Autodesk Inventor part; units mm, degrees
(part 2 of 2)
sketch "Sketch10" plane through (0, 0, 10) normal (0, 0, 1) x (1, 0, 0)
  arc A0 (18.6863, 97.4304) -> (17.9083, 97.5423) centre (18.2533, 97.1804) ccw projected
  line L0 (18.6863, 97.4304) -> (19.3213, 96.3305) projected
  arc A1 (19.3213, 96.3305) -> (21.9194, 97.8305) centre (20.6203, 97.0805) ccw projected
  line L1 (21.9194, 97.8305) -> (20.5344, 100.2294) projected
  line L2 (17.725, 88.9676) -> (14.955, 88.9676) projected
  arc A2 (14.955, 89.9676) -> (14.955, 88.9676) centre (14.955, 89.4676) ccw projected
  line L3 (14.955, 89.9676) -> (16.225, 89.9676) projected
  arc A3 (16.225, 89.9676) -> (17.6107, 92.0419) centre (16.225, 91.4676) ccw projected
  line L4 (19.6683, 99.7294) -> (21.0533, 97.3305) projected
  arc A4 (20.1873, 96.8305) -> (21.0533, 97.3305) centre (20.6203, 97.0805) ccw projected
  line L5 (20.1873, 96.8305) -> (19.5523, 97.9304) projected
  arc A5 (19.5523, 97.9304) -> (17.063, 98.0932) centre (18.2533, 97.1804) ccw projected
  arc A6 (11.8587, 96.3305) -> (12.1508, 95.6008) centre (12.2917, 96.0805) ccw projected
  line L6 (11.8587, 96.3305) -> (12.4937, 97.4304) projected
  arc A7 (12.4937, 97.4304) -> (9.8956, 98.9304) centre (11.1947, 98.1804) ccw projected
  line L7 (9.8956, 98.9304) -> (8.5106, 96.5315) projected
  arc A8 (16.225, 90.9676) -> (16.7109, 91.5854) centre (16.225, 91.4676) ccw projected
  line L8 (16.225, 90.9676) -> (14.955, 90.9676) projected
  arc A9 (14.955, 90.9676) -> (14.955, 87.9676) centre (14.955, 89.4676) ccw projected
  line L9 (14.955, 87.9676) -> (17.725, 87.9676) projected
  line L10 (9.3767, 96.0315) -> (10.7617, 98.4304) projected
  arc A10 (11.6277, 97.9304) -> (10.7617, 98.4304) centre (11.1947, 98.1804) ccw projected
  line L11 (11.6277, 97.9304) -> (10.9927, 96.8305) projected
  arc A11 (10.9927, 96.8305) -> (12.0963, 94.5933) centre (12.2917, 96.0805) ccw projected
  arc A12 (37.3863, 97.4304) -> (36.6083, 97.5423) centre (36.9533, 97.1804) ccw projected
  line L12 (37.3863, 97.4304) -> (38.0213, 96.3305) projected
  arc A13 (38.0213, 96.3305) -> (40.6194, 97.8305) centre (39.3203, 97.0805) ccw projected
  line L13 (40.6194, 97.8305) -> (39.2344, 100.2294) projected
  line L14 (36.425, 88.9676) -> (33.655, 88.9676) projected
  arc A14 (33.655, 89.9676) -> (33.655, 88.9676) centre (33.655, 89.4676) ccw projected
  line L15 (33.655, 89.9676) -> (34.925, 89.9676) projected
  arc A15 (34.925, 89.9676) -> (36.3107, 92.0419) centre (34.925, 91.4676) ccw projected
  line L16 (38.3683, 99.7294) -> (39.7533, 97.3305) projected
  arc A16 (38.8873, 96.8305) -> (39.7533, 97.3305) centre (39.3203, 97.0805) ccw projected
  line L17 (38.8873, 96.8305) -> (38.2523, 97.9304) projected
  arc A17 (38.2523, 97.9304) -> (35.763, 98.0932) centre (36.9533, 97.1804) ccw projected
  arc A18 (30.5587, 96.3305) -> (30.8508, 95.6008) centre (30.9917, 96.0805) ccw projected
  line L18 (30.5587, 96.3305) -> (31.1937, 97.4304) projected
  arc A19 (31.1937, 97.4304) -> (28.5956, 98.9304) centre (29.8947, 98.1804) ccw projected
  line L19 (28.5956, 98.9304) -> (27.2106, 96.5315) projected
  arc A20 (34.925, 90.9676) -> (35.4109, 91.5854) centre (34.925, 91.4676) ccw projected
  line L20 (34.925, 90.9676) -> (33.655, 90.9676) projected
  arc A21 (33.655, 90.9676) -> (33.655, 87.9676) centre (33.655, 89.4676) ccw projected
  line L21 (33.655, 87.9676) -> (36.425, 87.9676) projected
  line L22 (28.0767, 96.0315) -> (29.4617, 98.4304) projected
  arc A22 (30.3277, 97.9304) -> (29.4617, 98.4304) centre (29.8947, 98.1804) ccw projected
  line L23 (30.3277, 97.9304) -> (29.6927, 96.8305) projected
  arc A23 (29.6927, 96.8305) -> (30.7963, 94.5933) centre (30.9917, 96.0805) ccw projected
  arc A24 (56.0863, 97.4304) -> (55.3083, 97.5423) centre (55.6533, 97.1804) ccw projected
  line L24 (56.0863, 97.4304) -> (56.7213, 96.3305) projected
  arc A25 (56.7213, 96.3305) -> (59.3194, 97.8305) centre (58.0203, 97.0805) ccw projected
  line L25 (59.3194, 97.8305) -> (57.9344, 100.2294) projected
  line L26 (55.125, 88.9676) -> (52.355, 88.9676) projected
  arc A26 (52.355, 89.9676) -> (52.355, 88.9676) centre (52.355, 89.4676) ccw projected
  line L27 (52.355, 89.9676) -> (53.625, 89.9676) projected
  arc A27 (53.625, 89.9676) -> (55.0107, 92.0419) centre (53.625, 91.4676) ccw projected
  line L28 (57.0683, 99.7294) -> (58.4533, 97.3305) projected
  arc A28 (57.5873, 96.8305) -> (58.4533, 97.3305) centre (58.0203, 97.0805) ccw projected
  line L29 (57.5873, 96.8305) -> (56.9523, 97.9304) projected
  arc A29 (56.9523, 97.9304) -> (54.463, 98.0932) centre (55.6533, 97.1804) ccw projected
  arc A30 (49.2587, 96.3305) -> (49.5508, 95.6008) centre (49.6917, 96.0805) ccw projected
  line L30 (49.2587, 96.3305) -> (49.8937, 97.4304) projected
  arc A31 (49.8937, 97.4304) -> (47.2956, 98.9304) centre (48.5947, 98.1804) ccw projected
  line L31 (47.2956, 98.9304) -> (45.9106, 96.5315) projected
  arc A32 (53.625, 90.9676) -> (54.1109, 91.5854) centre (53.625, 91.4676) ccw projected
  line L32 (53.625, 90.9676) -> (52.355, 90.9676) projected
  arc A33 (52.355, 90.9676) -> (52.355, 87.9676) centre (52.355, 89.4676) ccw projected
  line L33 (52.355, 87.9676) -> (55.125, 87.9676) projected
  line L34 (46.7767, 96.0315) -> (48.1617, 98.4304) projected
  arc A34 (49.0277, 97.9304) -> (48.1617, 98.4304) centre (48.5947, 98.1804) ccw projected
  line L35 (49.0277, 97.9304) -> (48.3927, 96.8305) projected
  arc A35 (48.3927, 96.8305) -> (49.4963, 94.5933) centre (49.6917, 96.0805) ccw projected
  arc A36 (18.6863, 81.2704) -> (17.9083, 81.3823) centre (18.2533, 81.0204) ccw projected
  line L36 (18.6863, 81.2704) -> (19.3213, 80.1705) projected
  arc A37 (19.3213, 80.1705) -> (21.9194, 81.6705) centre (20.6203, 80.9205) ccw projected
  line L37 (21.9194, 81.6705) -> (20.5344, 84.0694) projected
  line L38 (17.725, 72.8076) -> (14.955, 72.8076) projected
  arc A38 (14.955, 73.8076) -> (14.955, 72.8076) centre (14.955, 73.3076) ccw projected
  line L39 (14.955, 73.8076) -> (16.225, 73.8076) projected
  arc A39 (16.225, 73.8076) -> (17.6107, 75.8819) centre (16.225, 75.3076) ccw projected
  line L40 (19.6683, 83.5694) -> (21.0533, 81.1705) projected
  arc A40 (20.1873, 80.6705) -> (21.0533, 81.1705) centre (20.6203, 80.9205) ccw projected
  line L41 (20.1873, 80.6705) -> (19.5523, 81.7704) projected
  arc A41 (19.5523, 81.7704) -> (17.063, 81.9332) centre (18.2533, 81.0204) ccw projected
  arc A42 (11.8587, 80.1705) -> (12.1508, 79.4408) centre (12.2917, 79.9205) ccw projected
  line L42 (11.8587, 80.1705) -> (12.4937, 81.2704) projected
  arc A43 (12.4937, 81.2704) -> (9.8956, 82.7704) centre (11.1947, 82.0204) ccw projected
  line L43 (9.8956, 82.7704) -> (8.5106, 80.3715) projected
  arc A44 (16.225, 74.8076) -> (16.7109, 75.4254) centre (16.225, 75.3076) ccw projected
  line L44 (16.225, 74.8076) -> (14.955, 74.8076) projected
  arc A45 (14.955, 74.8076) -> (14.955, 71.8076) centre (14.955, 73.3076) ccw projected
  line L45 (14.955, 71.8076) -> (17.725, 71.8076) projected
  line L46 (9.3767, 79.8715) -> (10.7617, 82.2704) projected
  arc A46 (11.6277, 81.7704) -> (10.7617, 82.2704) centre (11.1947, 82.0204) ccw projected
  line L47 (11.6277, 81.7704) -> (10.9927, 80.6705) projected
  arc A47 (10.9927, 80.6705) -> (12.0963, 78.4333) centre (12.2917, 79.9205) ccw projected
  arc A48 (37.3863, 81.2704) -> (36.6083, 81.3823) centre (36.9533, 81.0204) ccw projected
  line L48 (37.3863, 81.2704) -> (38.0213, 80.1705) projected
  arc A49 (38.0213, 80.1705) -> (40.6194, 81.6705) centre (39.3203, 80.9205) ccw projected
  line L49 (40.6194, 81.6705) -> (39.2344, 84.0694) projected
  line L50 (36.425, 72.8076) -> (33.655, 72.8076) projected
  arc A50 (33.655, 73.8076) -> (33.655, 72.8076) centre (33.655, 73.3076) ccw projected
  line L51 (33.655, 73.8076) -> (34.925, 73.8076) projected
  arc A51 (34.925, 73.8076) -> (36.3107, 75.8819) centre (34.925, 75.3076) ccw projected
  line L52 (38.3683, 83.5694) -> (39.7533, 81.1705) projected
  arc A52 (38.8873, 80.6705) -> (39.7533, 81.1705) centre (39.3203, 80.9205) ccw projected
  line L53 (38.8873, 80.6705) -> (38.2523, 81.7704) projected
  arc A53 (38.2523, 81.7704) -> (35.763, 81.9332) centre (36.9533, 81.0204) ccw projected
  arc A54 (30.5587, 80.1705) -> (30.8508, 79.4408) centre (30.9917, 79.9205) ccw projected
  line L54 (30.5587, 80.1705) -> (31.1937, 81.2704) projected
  arc A55 (31.1937, 81.2704) -> (28.5956, 82.7704) centre (29.8947, 82.0204) ccw projected
  line L55 (28.5956, 82.7704) -> (27.2106, 80.3715) projected
  arc A56 (34.925, 74.8076) -> (35.4109, 75.4254) centre (34.925, 75.3076) ccw projected
  line L56 (34.925, 74.8076) -> (33.655, 74.8076) projected
  arc A57 (33.655, 74.8076) -> (33.655, 71.8076) centre (33.655, 73.3076) ccw projected
  line L57 (33.655, 71.8076) -> (36.425, 71.8076) projected
  line L58 (28.0767, 79.8715) -> (29.4617, 82.2704) projected
  arc A58 (30.3277, 81.7704) -> (29.4617, 82.2704) centre (29.8947, 82.0204) ccw projected
  line L59 (30.3277, 81.7704) -> (29.6927, 80.6705) projected
  arc A59 (29.6927, 80.6705) -> (30.7963, 78.4333) centre (30.9917, 79.9205) ccw projected
  line L60 (46.7767, 79.8715) -> (48.1617, 82.2704) projected
  arc A60 (49.0277, 81.7704) -> (48.1617, 82.2704) centre (48.5947, 82.0204) ccw projected
  line L61 (49.0277, 81.7704) -> (48.3927, 80.6705) projected
  arc A61 (48.3927, 80.6705) -> (49.4963, 78.4333) centre (49.6917, 79.9205) ccw projected
  arc A62 (53.625, 74.8076) -> (54.1109, 75.4254) centre (53.625, 75.3076) ccw projected
  line L62 (53.625, 74.8076) -> (52.355, 74.8076) projected
  arc A63 (52.355, 74.8076) -> (52.355, 71.8076) centre (52.355, 73.3076) ccw projected
  line L63 (52.355, 71.8076) -> (55.125, 71.8076) projected
  line L64 (55.125, 72.8076) -> (52.355, 72.8076) projected
  arc A64 (52.355, 73.8076) -> (52.355, 72.8076) centre (52.355, 73.3076) ccw projected
  line L65 (52.355, 73.8076) -> (53.625, 73.8076) projected
  arc A65 (53.625, 73.8076) -> (55.0107, 75.8819) centre (53.625, 75.3076) ccw projected
  arc A66 (56.0863, 81.2704) -> (55.3083, 81.3823) centre (55.6533, 81.0204) ccw projected
  line L66 (56.0863, 81.2704) -> (56.7213, 80.1705) projected
  arc A67 (56.7213, 80.1705) -> (59.3194, 81.6705) centre (58.0203, 80.9205) ccw projected
  line L67 (59.3194, 81.6705) -> (57.9344, 84.0694) projected
  line L68 (57.0683, 83.5694) -> (58.4533, 81.1705) projected
  arc A68 (57.5873, 80.6705) -> (58.4533, 81.1705) centre (58.0203, 80.9205) ccw projected
  line L69 (57.5873, 80.6705) -> (56.9523, 81.7704) projected
  arc A69 (56.9523, 81.7704) -> (54.463, 81.9332) centre (55.6533, 81.0204) ccw projected
  arc A70 (49.2587, 80.1705) -> (49.5508, 79.4408) centre (49.6917, 79.9205) ccw projected
  line L70 (49.2587, 80.1705) -> (49.8937, 81.2704) projected
  arc A71 (49.8937, 81.2704) -> (47.2956, 82.7704) centre (48.5947, 82.0204) ccw projected
  line L71 (47.2956, 82.7704) -> (45.9106, 80.3715) projected
  circle A72 centre (34.29, 35.56) radius 30.149 projected
  circle A73 centre (25.4912, 73.6695) radius 2.55 projected
  circle A74 centre (44.1912, 73.6695) radius 2.55 projected
  circle A75 centre (6.7912, 73.6695) radius 2.55 projected
  line L72 (63.58, 2) -> (5, 2) projected
  arc A76 (63.58, 2) -> (66.58, 5) centre (63.58, 5) ccw projected
  line L73 (66.58, 102.95) -> (66.58, 5) projected
  arc A77 (66.58, 102.95) -> (63.58, 105.95) centre (63.58, 102.95) ccw projected
  line L74 (5, 105.95) -> (63.58, 105.95) projected
  arc A78 (5, 105.95) -> (2, 102.95) centre (5, 102.95) ccw projected
  line L75 (2, 5) -> (2, 102.95) projected
  arc A79 (2, 5) -> (5, 2) centre (5, 5) ccw projected
  arc A80 (17.063, 98.0932) -> (12.1508, 95.6008) centre (15.59, 94.9095) ccw projected
  line L76 (17.725, 87.9676) -> (17.725, 86.9676) projected
  line L77 (17.725, 86.9676) -> (14.955, 86.9676) projected
  arc A81 (12.6621, 88.4712) -> (14.955, 86.9676) centre (14.955, 89.4676) ccw projected
  line L78 (8.5106, 96.5315) -> (7.6446, 97.0315) projected
  line L79 (7.6446, 97.0315) -> (9.0296, 99.4304) projected
  arc A82 (11.4782, 100.6643) -> (9.0296, 99.4304) centre (11.1947, 98.1804) ccw projected
  line L80 (20.5344, 100.2294) -> (21.4004, 100.7294) projected
  line L81 (21.4004, 100.7294) -> (22.7854, 98.3305) projected
  arc A83 (22.6297, 95.5931) -> (22.7854, 98.3305) centre (20.6203, 97.0805) ccw projected
  arc A84 (35.763, 98.0932) -> (30.8508, 95.6008) centre (34.29, 94.9095) ccw projected
  line L82 (36.425, 87.9676) -> (36.425, 86.9676) projected
  line L83 (36.425, 86.9676) -> (33.655, 86.9676) projected
  arc A85 (31.3621, 88.4712) -> (33.655, 86.9676) centre (33.655, 89.4676) ccw projected
  line L84 (27.2106, 96.5315) -> (26.3446, 97.0315) projected
  line L85 (26.3446, 97.0315) -> (27.7296, 99.4304) projected
  arc A86 (30.1782, 100.6643) -> (27.7296, 99.4304) centre (29.8947, 98.1804) ccw projected
  line L86 (39.2344, 100.2294) -> (40.1004, 100.7294) projected
  line L87 (40.1004, 100.7294) -> (41.4854, 98.3305) projected
  arc A87 (41.3297, 95.5931) -> (41.4854, 98.3305) centre (39.3203, 97.0805) ccw projected
  arc A88 (54.463, 98.0932) -> (49.5508, 95.6008) centre (52.99, 94.9095) ccw projected
  line L88 (55.125, 87.9676) -> (55.125, 86.9676) projected
  line L89 (55.125, 86.9676) -> (52.355, 86.9676) projected
  arc A89 (50.0621, 88.4712) -> (52.355, 86.9676) centre (52.355, 89.4676) ccw projected
  line L90 (45.9106, 96.5315) -> (45.0446, 97.0315) projected
  line L91 (45.0446, 97.0315) -> (46.4296, 99.4304) projected
  arc A90 (48.8782, 100.6643) -> (46.4296, 99.4304) centre (48.5947, 98.1804) ccw projected
  line L92 (57.9344, 100.2294) -> (58.8004, 100.7294) projected
  line L93 (58.8004, 100.7294) -> (60.1854, 98.3305) projected
  arc A91 (60.0297, 95.5931) -> (60.1854, 98.3305) centre (58.0203, 97.0805) ccw projected
  arc A92 (17.063, 81.9332) -> (12.1508, 79.4408) centre (15.59, 78.7495) ccw projected
  line L94 (17.725, 71.8076) -> (17.725, 70.8076) projected
  line L95 (17.725, 70.8076) -> (14.955, 70.8076) projected
  arc A93 (12.6621, 72.3112) -> (14.955, 70.8076) centre (14.955, 73.3076) ccw projected
  line L96 (8.5106, 80.3715) -> (7.6446, 80.8715) projected
  line L97 (7.6446, 80.8715) -> (9.0296, 83.2704) projected
  arc A94 (11.4782, 84.5043) -> (9.0296, 83.2704) centre (11.1947, 82.0204) ccw projected
  line L98 (20.5344, 84.0694) -> (21.4004, 84.5694) projected
  line L99 (21.4004, 84.5694) -> (22.7854, 82.1705) projected
  arc A95 (22.6297, 79.4331) -> (22.7854, 82.1705) centre (20.6203, 80.9205) ccw projected
  arc A96 (35.763, 81.9332) -> (30.8508, 79.4408) centre (34.29, 78.7495) ccw projected
  line L100 (36.425, 71.8076) -> (36.425, 70.8076) projected
  line L101 (36.425, 70.8076) -> (33.655, 70.8076) projected
  arc A97 (31.3621, 72.3112) -> (33.655, 70.8076) centre (33.655, 73.3076) ccw projected
  line L102 (27.2106, 80.3715) -> (26.3446, 80.8715) projected
  line L103 (26.3446, 80.8715) -> (27.7296, 83.2704) projected
  arc A98 (30.1782, 84.5043) -> (27.7296, 83.2704) centre (29.8947, 82.0204) ccw projected
  line L104 (39.2344, 84.0694) -> (40.1004, 84.5694) projected
  line L105 (40.1004, 84.5694) -> (41.4854, 82.1705) projected
  arc A99 (41.3297, 79.4331) -> (41.4854, 82.1705) centre (39.3203, 80.9205) ccw projected
  line L106 (55.125, 71.8076) -> (55.125, 70.8076) projected
  line L107 (55.125, 70.8076) -> (52.355, 70.8076) projected
  arc A100 (50.0621, 72.3112) -> (52.355, 70.8076) centre (52.355, 73.3076) ccw projected
  line L108 (45.9106, 80.3715) -> (45.0446, 80.8715) projected
  line L109 (45.0446, 80.8715) -> (46.4296, 83.2704) projected
  arc A101 (48.8782, 84.5043) -> (46.4296, 83.2704) centre (48.5947, 82.0204) ccw projected
  line L110 (57.9344, 84.0694) -> (58.8004, 84.5694) projected
  line L111 (58.8004, 84.5694) -> (60.1854, 82.1705) projected
  arc A102 (60.0297, 79.4331) -> (60.1854, 82.1705) centre (58.0203, 80.9205) ccw projected
  line L112 (11.4782, 100.6643) -> (19.6683, 99.7294) projected
  arc A103 (17.6107, 92.0419) -> (17.9083, 97.5423) centre (15.59, 94.9095) ccw projected
  line L113 (22.6297, 95.5931) -> (17.725, 88.9676) projected
  line L114 (30.1782, 100.6643) -> (38.3683, 99.7294) projected
  arc A104 (36.3107, 92.0419) -> (36.6083, 97.5423) centre (34.29, 94.9095) ccw projected
  line L115 (41.3297, 95.5931) -> (36.425, 88.9676) projected
  line L116 (48.8782, 100.6643) -> (57.0683, 99.7294) projected
  arc A105 (55.0107, 92.0419) -> (55.3083, 97.5423) centre (52.99, 94.9095) ccw projected
  line L117 (60.0297, 95.5931) -> (55.125, 88.9676) projected
  line L118 (11.4782, 84.5043) -> (19.6683, 83.5694) projected
  arc A106 (17.6107, 75.8819) -> (17.9083, 81.3823) centre (15.59, 78.7495) ccw projected
  line L119 (22.6297, 79.4331) -> (17.725, 72.8076) projected
  line L120 (30.1782, 84.5043) -> (38.3683, 83.5694) projected
  arc A107 (36.3107, 75.8819) -> (36.6083, 81.3823) centre (34.29, 78.7495) ccw projected
  line L121 (41.3297, 79.4331) -> (36.425, 72.8076) projected
  arc A108 (12.0963, 94.5933) -> (16.7109, 91.5854) centre (15.59, 94.9095) ccw projected
  line L122 (12.6621, 88.4712) -> (9.3767, 96.0315) projected
  arc A109 (30.7963, 94.5933) -> (35.4109, 91.5854) centre (34.29, 94.9095) ccw projected
  line L123 (31.3621, 88.4712) -> (28.0767, 96.0315) projected
  arc A110 (49.4963, 94.5933) -> (54.1109, 91.5854) centre (52.99, 94.9095) ccw projected
  line L124 (50.0621, 88.4712) -> (46.7767, 96.0315) projected
  arc A111 (12.0963, 78.4333) -> (16.7109, 75.4254) centre (15.59, 78.7495) ccw projected
  line L125 (12.6621, 72.3112) -> (9.3767, 79.8715) projected
  arc A112 (30.7963, 78.4333) -> (35.4109, 75.4254) centre (34.29, 78.7495) ccw projected
  line L126 (31.3621, 72.3112) -> (28.0767, 79.8715) projected
  arc A113 (54.463, 81.9332) -> (49.5508, 79.4408) centre (52.99, 78.7495) ccw projected
  line L127 (48.8782, 84.5043) -> (57.0683, 83.5694) projected
  arc A114 (55.0107, 75.8819) -> (55.3083, 81.3823) centre (52.99, 78.7495) ccw projected
  line L128 (60.0297, 79.4331) -> (55.125, 72.8076) projected
  line L129 (50.0621, 72.3112) -> (46.7767, 79.8715) projected
  arc A115 (49.4963, 78.4333) -> (54.1109, 75.4254) centre (52.99, 78.7495) ccw projected
  point P0 (0, 0)
hole "Hole1" at (5, 102.95, 10) at (63.58, 102.95, 10) at (63.58, 5, 10) at (5, 5, 10) direction (0, 0, -1) diameter 3.4036 end through all clearance for "Flat Head Machine Screw" size "M3" standard "Ansi Metric M Profile"
sketch "Sketch11" plane through (0, 0, 0) normal (0, 0, -1) x (-1, 0, 0)
  circle A0 centre (-63.58, 5) radius 1.7018 projected
  circle A1 centre (-5, 5) radius 1.7018 projected
  circle A2 centre (-56.2991, 22.853) radius 2 projected
  circle A3 centre (-12.2809, 22.853) radius 2 projected
  circle A4 centre (-34.29, 60.9739) radius 2 projected
  circle A5 centre (-34.29, 35.56) radius 21.3606 projected
  line L0 (-3, 104.95) -> (-3, 66.587) projected
  line L1 (-3, 66.587) -> (-65.58, 66.587) projected
  line L2 (-65.58, 66.587) -> (-65.58, 104.95) projected
  line L3 (-65.58, 104.95) -> (-3, 104.95) projected
  arc A6 (-68.58, 5) -> (-63.58, 0) centre (-63.58, 5) ccw projected
  line L4 (-5, 0) -> (-63.58, 0) projected
  arc A7 (-5, 0) -> (0, 5) centre (-5, 5) ccw projected
  line L5 (0, 102.95) -> (0, 5) projected
  arc A8 (0, 102.95) -> (-5, 107.95) centre (-5, 102.95) ccw projected
  line L6 (-63.58, 107.95) -> (-5, 107.95) projected
  arc A9 (-63.58, 107.95) -> (-68.58, 102.95) centre (-63.58, 102.95) ccw projected
  line L7 (-68.58, 5) -> (-68.58, 102.95) projected
  line L8 (-65.58, 63.587) -> (-2, 63.587)
  line L9 (-65.58, 63.587) -> (-65.58, 2)
  circle A10 centre (-63.58, 5) radius 4.7018
  line L10 (-2, 63.587) -> (-2, 2)
  line L11 (-2, 2) -> (-65.58, 2)
  circle A11 centre (-5, 5) radius 4.7018
  circle A12 centre (-34.29, 60.9739) radius 5
  circle A13 centre (-12.2809, 22.853) radius 5
  circle A14 centre (-56.2991, 22.853) radius 5
  line L12 (-66.58, 102.95) -> (-66.58, 5) projected
  arc A15 (-66.58, 12.7018) -> (-63.58, 9.7018) centre (-63.58, 12.7018) ccw
  arc A16 (-58.8782, 5) -> (-55.8782, 2) centre (-55.8782, 5) ccw
  arc A17 (-12.7018, 2) -> (-9.7018, 5) centre (-12.7018, 5) ccw
  arc A18 (-5, 9.7018) -> (-2, 12.7018) centre (-5, 12.7018) ccw
  circle A19 centre (-34.29, 60.9739) radius 2 projected
  circle A20 centre (-56.2991, 22.853) radius 2 projected
  circle A21 centre (-12.2809, 22.853) radius 2 projected
  circle A22 centre (-34.29, 60.9739) radius 2 projected
  circle A23 centre (-34.29, 35.56) radius 30.149 projected
  circle A24 centre (-34.29, 35.56) radius 21.3606 projected
  circle A25 centre (-34.29, 35.56) radius 32.649
  point P0 (0, 0)
  point P1 (-66.58, 70.9374)
  point P2 (-66.58, 100.95)
  point P3 (-2, 30.7316)
  point P4 (-27.9749, 2)
  point P5 (-40.6051, 2)
  point P6 (-65.58, 26.2384)
  point P7 (-65.58, 10.4657)
  point P8 (-65.58, 44.8816)
  point P9 (-51.0365, 63.587)
  point P10 (-17.5435, 63.587)
  point P11 (-2, 40.3884)
  point P12 (-2, 8.6203)
  point P13 (-8.6203, 2)
  point P14 (-59.9597, 2)
  point P15 (-65.58, 9.2552)
  dimension "d105" = 3
  dimension "d107" = 3
  dimension "d109" = 3
  dimension "d110" = 3
  dimension "d111" = 3
  dimension "d112" = 3
  dimension "d113" = 3
  dimension "d114" = 3
  dimension "d115" = 2
  dimension "d116" = 2
  dimension "d118" = 2.5
  constraints: 12 point on circle, 10 centre point, 7 tangent, 6 end point, 3 horizontal, 3 point on line, 2 equal radius, 2 vertical alignment, 1 perpendicular, 6 other
  measures "d105" distance between parallel lines of L7 L2
  measures "d107" distance between parallel lines of L1 L8
  measures "d110" radial gap between concentric circles of A10 A0
  measures "d111" radial gap between concentric circles of A1 A11
  measures "d112" radial gap between concentric circles of A4 A12
  measures "d113" radial gap between concentric circles of A3 A13
  measures "d114" radial gap between concentric circles of A2 A14
  measures "d115" distance between parallel lines of L4 L11
  measures "d116" distance between parallel lines of L5 L10
  measures "d118" radial gap between concentric circles of A23 A25
extrude "Extrusion12" cut sketch "Sketch11" against normal blind 8 contours A25 L9 L8 | L8 L10 A25 | A25 L10 A18 A11 A17 L11 A16 A10 A15 L9
fillet "Fillet2" radius 1 6 edges at (17.5435, 63.587, 4) (51.0365, 63.587, 4) (2, 40.3884, 4) (2, 30.7316, 4) (65.58, 44.8816, 4) (65.58, 26.2384, 4)
fillet "Fillet3" radius 5 2 edges at (65.58, 63.587, 4) (2, 63.587, 4)
fillet "Fillet4" radius 3 2 edges at (65.58, 66.587, 2.05) (3, 66.587, 2.05)
sketch "Sketch12" plane through (0, 0, 4.1) normal (0, 0, -1) x (-1, 0, 0)
  circle A0 centre (-63.58, 102.95) radius 1.7018 projected
  circle A1 centre (-63.58, 102.95) radius 4.7018
  circle A2 centre (-5, 102.95) radius 1.7018 projected
  circle A3 centre (-5, 102.95) radius 4.7018
  arc A4 (-9.7018, 102.95) -> (-11.7018, 104.95) centre (-11.7018, 102.95) ccw
  arc A5 (-3, 96.2482) -> (-5, 98.2482) centre (-5, 96.2482) ccw
  line L0 (-65.58, 104.95) -> (-3, 104.95) projected
  line L1 (-3, 104.95) -> (-3, 66.587) projected
  arc A6 (-56.8782, 104.95) -> (-58.8782, 102.95) centre (-56.8782, 102.95) ccw
  arc A7 (-63.58, 98.2482) -> (-65.58, 96.2482) centre (-63.58, 96.2482) ccw
  line L2 (-65.58, 66.587) -> (-65.58, 104.95) projected
  point P0 (0, 0)
  point P1 (-63.58, 105.95)
  point P2 (-5, 105.95)
  point P3 (-2, 102.95)
  point P4 (-3, 69.587)
  point P5 (-65.58, 69.587)
  point P6 (-66.58, 102.95)
  point P7 (-8.6203, 105.95)
  point P8 (-2, 99.3297)
  point P9 (-59.9597, 105.95)
  point P10 (-66.58, 99.3297)
  point P11 (-3, 66.587)
  point P12 (-3, 98.6948)
  point P13 (-9.2552, 104.95)
  point P14 (-65.58, 98.6948)
  point P15 (-59.3248, 104.95)
  dimension "d124" = 3
  dimension "d125" = 3
  constraints: 12 point on circle, 6 centre point, 4 tangent, 3 equal radius, 1 horizontal alignment, 11 other
  measures "d124" radial gap between concentric circles of A0 A1
  measures "d125" radial gap between concentric circles of A2 A3
extrude "Extrusion13" add sketch "Sketch12" along normal up to surface (4.1 mm away) contours A1 L2 L0 | A7 L2 A1 | A1 L0 A6 | A3 L0 L1 | A4 L0 A3 | A3 L1 A5 picked at (-59.9175, 102.6013) picked at (-8.6625, 102.6013)
equation "\"d17\" = d16"
body "Solid1"
